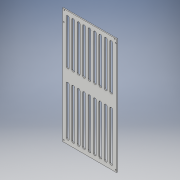
# Autodesk Inventor part: GlyphPlateUnderside
Saved by Autodesk Inventor 2017 (Build 210142000, 142)
## iProperties
Created: 2018-01-27
Part Number: GlyphPlateUnderside
Material: Generic
Document SubType Name: Modeling
Designer: User
Density: 1 g/cm^3
Appearance: Default
Author: User
Autodesk Inventor part; units mm, degrees
ref_plane "YZ Plane" through (0, 0, 0) normal (1, 0, 0) x (0, 1, 0)
ref_plane "XZ Plane" through (0, 0, 0) normal (0, 1, 0) x (-1, 0, 0)
ref_plane "XY Plane" through (0, 0, 0) normal (0, 0, 1) x (1, 0, 0)
sketch "Sketch1" plane through (0, 0, 0) normal (0, 0, 1) x (1, 0, 0)
  line L0 (0, 0) -> (178.2064, 0)
  line L1 (178.2064, 0) -> (178.2064, 381)
  line L2 (178.2064, 381) -> (0, 381)
  line L3 (0, 381) -> (0, 0)
  dimension "d0" = 178.2064
  dimension "d1" = 381
  constraints: 8 end point, 2 parallel, 1 horizontal, 1 perpendicular
  measures "d0" distance of L2.end L1.end
  measures "d1" distance of L1.end L0.end
extrude "Extrusion1" add sketch "Sketch1" along normal blind 3.175
sketch "Sketch2" plane through (0, 0, 3.175) normal (0, 0, 1) x (1, 0, 0)
  line L0 (0, 0) -> (178.2064, 0) projected
  line L1 (0, 0) -> (4.0386, 0)
  line L2 (4.0386, 0) -> (4.0386, 6.35)
  line L3 (0, 381) -> (0, 0) projected
  line L4 (0, 381) -> (4.0386, 381)
  line L5 (178.2064, 381) -> (0, 381) projected
  line L6 (4.0386, 381) -> (4.0386, 342.9)
  line L7 (4.0386, 381) -> (42.1386, 381) construction
  line L8 (0, 381) -> (0, 377.825)
  line L9 (0, 377.825) -> (6.35, 377.825)
  line L10 (178.2064, 0) -> (178.2064, 381) projected
  line L11 (178.2064, 0) -> (175.0314, 0)
  line L12 (175.0314, 0) -> (175.0314, 6.35)
  line L13 (178.2064, 377.825) -> (171.8564, 377.825)
  point P0 (175.0314, 368.3)
  dimension "d4" = 4.0386
  dimension "d5" = 6.35
  dimension "d6" = 38.1
  dimension "d7" = 90
  dimension "d8" = 3.175
  dimension "d9" = 6.35
  dimension "d10" = 3.175
  dimension "d11" = 6.35
  dimension "d19" = 4.0386
  dimension "d21" = 3.175
  dimension "d22" = 12.7
  dimension "d23" = 3.175
  constraints: 20 end point, 5 coincident, 5 perpendicular, 5 point on line, 1 horizontal, 1 vertical
  measures "d4" distance of L0.start L1.end
  measures "d5" distance of L1.end L2.end
  measures "d6" distance of L4.end L6.end
  measures "d7" angle of L6 L7
  measures "d8" distance of L3.start L8.end
  measures "d9" distance of L8.end L9.end
  measures "d10" distance of L0.end L11.end
  measures "d11" distance of L13.start L13.end
  measures "d19" distance between parallel lines of L3 L6
  measures "d21" distance from line of L10 point (175.031, 368.3)
  measures "d22" distance from line of point (175.031, 368.3) L5
  measures "d23" distance from line of L5 L13.end
hole "Hole1" at (4.0386, 6.35, 3.175) at (4.0386, 342.9, 3.175) at (6.35, 377.825, 3.175) at (175.0314, 6.35, 3.175) at (175.0314, 368.3, 3.175) at (171.8564, 377.825, 3.175) direction (0, 0, -1) diameter 3.556 depth 25.4 tip angle 118
sketch "Sketch3" plane through (0, 0, 3.175) normal (0, 0, 1) x (1, 0, 0)
  line L0 (17.4625, 12.7) -> (17.4625, 177.8) construction
  line L1 (22.225, 17.4625) -> (22.225, 173.0375)
  line L2 (12.7, 173.0375) -> (12.7, 17.4625)
  arc A0 (12.7, 17.4625) -> (22.225, 17.4625) centre (17.4625, 17.4625) ccw
  arc A1 (22.225, 173.0375) -> (12.7, 173.0375) centre (17.4625, 173.0375) ccw
  line L3 (0, 381) -> (0, 0) projected
  line L4 (178.2064, 0) -> (178.2064, 381) projected
  line L5 (0, 0) -> (178.2064, 0) projected
  line L6 (35.3695, 12.7) -> (35.3695, 177.8) construction
  line L7 (40.132, 17.4625) -> (40.132, 173.0375)
  line L8 (30.607, 173.0375) -> (30.607, 17.4625)
  arc A2 (30.607, 17.4625) -> (40.132, 17.4625) centre (35.3695, 17.4625) ccw
  arc A3 (40.132, 173.0375) -> (30.607, 173.0375) centre (35.3695, 173.0375) ccw
  line L9 (53.2765, 12.7) -> (53.2765, 177.8) construction
  line L10 (58.039, 17.4625) -> (58.039, 173.0375)
  line L11 (48.514, 173.0375) -> (48.514, 17.4625)
  arc A4 (48.514, 17.4625) -> (58.039, 17.4625) centre (53.2765, 17.4625) ccw
  arc A5 (58.039, 173.0375) -> (48.514, 173.0375) centre (53.2765, 173.0375) ccw
  line L12 (71.1835, 12.7) -> (71.1835, 177.8) construction
  line L13 (75.946, 17.4625) -> (75.946, 173.0375)
  line L14 (66.421, 173.0375) -> (66.421, 17.4625)
  arc A6 (66.421, 17.4625) -> (75.946, 17.4625) centre (71.1835, 17.4625) ccw
  arc A7 (75.946, 173.0375) -> (66.421, 173.0375) centre (71.1835, 173.0375) ccw
  line L15 (89.0905, 12.7) -> (89.0905, 177.8) construction
  line L16 (93.853, 17.4625) -> (93.853, 173.0375)
  line L17 (84.328, 173.0375) -> (84.328, 17.4625)
  arc A8 (84.328, 17.4625) -> (93.853, 17.4625) centre (89.0905, 17.4625) ccw
  arc A9 (93.853, 173.0375) -> (84.328, 173.0375) centre (89.0905, 173.0375) ccw
  line L18 (106.9975, 12.7) -> (106.9975, 177.8) construction
  line L19 (111.76, 17.4625) -> (111.76, 173.0375)
  line L20 (102.235, 173.0375) -> (102.235, 17.4625)
  arc A10 (102.235, 17.4625) -> (111.76, 17.4625) centre (106.9975, 17.4625) ccw
  arc A11 (111.76, 173.0375) -> (102.235, 173.0375) centre (106.9975, 173.0375) ccw
  line L21 (124.9045, 12.7) -> (124.9045, 177.8) construction
  line L22 (129.667, 17.4625) -> (129.667, 173.0375)
  line L23 (120.142, 173.0375) -> (120.142, 17.4625)
  arc A12 (120.142, 17.4625) -> (129.667, 17.4625) centre (124.9045, 17.4625) ccw
  arc A13 (129.667, 173.0375) -> (120.142, 173.0375) centre (124.9045, 173.0375) ccw
  line L24 (142.8115, 12.7) -> (142.8115, 177.8) construction
  line L25 (147.574, 17.4625) -> (147.574, 173.0375)
  line L26 (138.049, 173.0375) -> (138.049, 17.4625)
  arc A14 (138.049, 17.4625) -> (147.574, 17.4625) centre (142.8115, 17.4625) ccw
  arc A15 (147.574, 173.0375) -> (138.049, 173.0375) centre (142.8115, 173.0375) ccw
  line L27 (160.7328, 14.2764) -> (160.7328, 166.6986) construction
  line L28 (165.5064, 19.05) -> (165.5064, 161.925)
  line L29 (155.9592, 161.925) -> (155.9592, 19.05)
  line L30 (160.7185, 12.7) -> (160.7185, 177.8) construction
  line L31 (165.481, 17.4625) -> (165.481, 173.0375)
  line L32 (155.956, 173.0375) -> (155.956, 17.4625)
  arc A16 (155.956, 17.4625) -> (165.481, 17.4625) centre (160.7185, 17.4625) ccw
  arc A17 (165.481, 173.0375) -> (155.956, 173.0375) centre (160.7185, 173.0375) ccw
  line L33 (178.2064, 0) -> (178.2064, 381) projected
  line L34 (17.4625, 368.3) -> (17.4625, 215.9) construction
  line L35 (22.225, 363.5375) -> (22.225, 220.6625)
  line L36 (12.7, 220.6625) -> (12.7, 363.5375)
  arc A18 (22.225, 363.5375) -> (12.7, 363.5375) centre (17.4625, 363.5375) ccw
  arc A19 (12.7, 220.6625) -> (22.225, 220.6625) centre (17.4625, 220.6625) ccw
  arc A20 (30.6102, 220.6625) -> (40.1352, 220.6625) centre (35.3727, 220.6625) ccw
  line L37 (40.1352, 363.5375) -> (40.1352, 220.6625)
  line L38 (30.6102, 220.6625) -> (30.6102, 363.5375)
  line L39 (35.3727, 368.3) -> (35.3727, 215.9) construction
  arc A21 (40.1352, 363.5375) -> (30.6102, 363.5375) centre (35.3727, 363.5375) ccw
  arc A22 (48.5204, 220.6625) -> (58.0453, 220.6625) centre (53.2829, 220.6625) ccw
  line L40 (58.0453, 363.5375) -> (58.0453, 220.6625)
  line L41 (48.5204, 220.6625) -> (48.5204, 363.5375)
  line L42 (53.2828, 368.3) -> (53.2829, 215.9) construction
  arc A23 (58.0453, 363.5375) -> (48.5204, 363.5375) centre (53.2828, 363.5375) ccw
  arc A24 (66.4305, 220.6625) -> (75.9555, 220.6625) centre (71.193, 220.6625) ccw
  line L43 (75.9555, 363.5375) -> (75.9555, 220.6625)
  line L44 (66.4305, 220.6625) -> (66.4305, 363.5375)
  line L45 (71.193, 368.3) -> (71.193, 215.9) construction
  arc A25 (75.9555, 363.5375) -> (66.4305, 363.5375) centre (71.193, 363.5375) ccw
  arc A26 (84.3407, 220.6625) -> (93.8657, 220.6625) centre (89.1032, 220.6625) ccw
  line L46 (93.8657, 363.5375) -> (93.8657, 220.6625)
  line L47 (84.3407, 220.6625) -> (84.3407, 363.5375)
  line L48 (89.1032, 368.3) -> (89.1032, 215.9) construction
  arc A27 (93.8657, 363.5375) -> (84.3407, 363.5375) centre (89.1032, 363.5375) ccw
  arc A28 (102.2509, 220.6625) -> (111.7759, 220.6625) centre (107.0134, 220.6625) ccw
  line L49 (111.7759, 363.5375) -> (111.7759, 220.6625)
  line L50 (102.2509, 220.6625) -> (102.2509, 363.5375)
  line L51 (107.0134, 368.3) -> (107.0134, 215.9) construction
  arc A29 (111.7759, 363.5375) -> (102.2509, 363.5375) centre (107.0134, 363.5375) ccw
  arc A30 (120.161, 220.6625) -> (129.686, 220.6625) centre (124.9236, 220.6625) ccw
  line L52 (129.686, 363.5375) -> (129.686, 220.6625)
  line L53 (120.161, 220.6625) -> (120.161, 363.5375)
  line L54 (124.9236, 368.3) -> (124.9236, 215.9) construction
  arc A31 (129.686, 363.5375) -> (120.161, 363.5375) centre (124.9236, 363.5375) ccw
  arc A32 (138.0712, 220.6625) -> (147.5962, 220.6625) centre (142.8337, 220.6625) ccw
  line L55 (147.5962, 363.5375) -> (147.5962, 220.6625)
  line L56 (138.0712, 220.6625) -> (138.0712, 363.5375)
  line L57 (142.8337, 368.3) -> (142.8337, 215.9) construction
  arc A33 (147.5962, 363.5375) -> (138.0712, 363.5375) centre (142.8337, 363.5375) ccw
  arc A34 (155.9814, 220.6625) -> (165.5064, 220.6625) centre (160.7439, 220.6625) ccw
  line L58 (165.5064, 363.5375) -> (165.5064, 220.6625)
  line L59 (155.9814, 220.6625) -> (155.9814, 363.5375)
  line L60 (160.7439, 368.3) -> (160.7439, 215.9) construction
  arc A35 (165.5064, 363.5375) -> (155.9814, 363.5375) centre (160.7439, 363.5375) ccw
  point P0 (17.4625, 95.25)
  point P1 (35.3695, 95.25)
  point P2 (53.2765, 95.25)
  point P3 (71.1835, 95.25)
  point P4 (89.0905, 95.25)
  point P5 (106.9975, 95.25)
  point P6 (124.9045, 95.25)
  point P7 (142.8115, 95.25)
  point P8 (144.4212, 90.4875)
  point P9 (160.7185, 95.25)
  point P10 (17.4625, 292.1)
  point P11 (35.3727, 292.1)
  point P12 (53.2829, 292.1)
  point P13 (71.193, 292.1)
  point P14 (89.1032, 292.1)
  point P15 (107.0134, 292.1)
  point P16 (124.9236, 292.1)
  point P17 (142.8337, 292.1)
  point P18 (160.7439, 292.1)
  dimension "d24" = 9.525
  dimension "d27" = 12.7
  dimension "d34" = 12.7
  dimension "d39" = 381
  dimension "d41" = 165.1
  dimension "d46" = 17.907
  dimension "d51" = 12.7
  dimension "d52" = 8.3852
  dimension "d55" = 17.9102
  constraints: 152 end point, 108 point on circle, 36 centre point, 36 point on line, 4 tangent, 2 horizontal, 1 midpoint, 1 parallel, 1 vertical, 224 other
  measures "d24" diameter of A1
  measures "d27" distance between parallel lines of L3 L2
  measures "d34" distance from line of L5 L0.start
  measures "d39" distance of L4.start L4.end
  measures "d41" distance of L0.start L0.end
  measures "d46" distance of L1.start L7.start
  measures "d51" distance between parallel lines of L4 L28
  measures "d52" distance between parallel lines of L25 L29
  measures "d55" distance of L34.end L39.end
extrude "Extrusion2" cut sketch "Sketch3" against normal through all
body "Solid1"
